pipe elements_v8 (Autodesk Fusion 360 design; units mm, degrees)
Autodesk Fusion 360 part; units mm, degrees
sketch "Esquisse1" plane through (0, 0, 0) normal (0, 0, 1) x (1, 0, 0) in component "part_1"
  circle A0 centre (0, 0) radius 12.5
  circle A1 centre (0, 0) radius 15.25
  circle A2 centre (0, 0) radius 13.5
  dimension "d1" = 25
  dimension "d2" = 30.5
  dimension "d3" = 1
  constraint coincident A0.centre A1.centre
  measures "d1" diameter of A0
  measures "d2" diameter of A1
extrude "Extrusion1" add sketch "Esquisse1" along normal blind 103 contours A2 makes body 1 in component "part_1"
extrude "Extrusion2" add sketch "Esquisse1" along normal blind 15 contours A1 bodies 1 in component "part_1"
sketch "Esquisse1 (2)" plane through (0, 0, 103) normal (0, 0, 1) x (-1, 0, 0) in component "part_2"
  circle A0 centre (0, 0) radius 12.5
  circle A1 centre (0, 0) radius 13.5
  circle A2 centre (0, 0) radius 12.5
  circle A3 centre (0, 0) radius 13.5
  circle A4 centre (0, 0) radius 15.25
extrude "Extrusion1'" add sketch "Esquisse1 (2)" along normal blind 100 separate body contours A1 A3 makes body 2 in component "part_2"
extrude "Extrusion2'" add sketch "Esquisse1 (2)" along normal blind 10 and the other way blind 10 contours A4 bodies 2 in component "part_2"
sketch "Esquisse1 (3)" plane through (0, 0, 203) normal (0, 0, 1) x (-1, 0, 0) in component "part_3"
  circle A0 centre (0, 0) radius 12.5
  circle A1 centre (0, 0) radius 13.5
  circle A2 centre (0, 0) radius 12.5
  circle A3 centre (0, 0) radius 13.5
  circle A4 centre (0, 0) radius 15.25
extrude "Extrusion1''" add sketch "Esquisse1 (3)" along normal blind 50 separate body contours A1 A3 makes body 3 in component "part_3"
extrude "Extrusion2''" add sketch "Esquisse1 (3)" along normal blind 10 and the other way blind 10 contours A4 bodies 3 in component "part_3"
sketch "Esquisse2" plane through (0, 0, 253) normal (0, 0, 1) x (-1, 0, 0) in component "part_3"
  circle A0 centre (0, 0) radius 12.5
  circle A1 centre (0, 0) radius 13.5
  circle A2 centre (0, 0) radius 15
  circle A3 centre (0, 0) radius 17
  dimension "d23" = 30
  dimension "d24" = 2
  constraint coincident A0.centre A1.centre
  measures "d23" diameter of A2
loft "Lissage1" add profiles "Esquisse2", "Esquisse1 (3)" section 1 contours A3 section 2 contours A1 A3 bodies 3 in component "part_3"
loft "Lissage2" cut profiles "Esquisse2", "Esquisse1 (3)" section 1 contours A0 | A1 | A2 section 2 contours A0 A2 bodies 3 in component "part_3"
chamfer "Chanfrein2" distance 1.75 angle 45 1 edges at (12.5864, 4.8818, 113) on bodies 2 in component "part_2"
chamfer "Chanfrein1" distance 1 angle 45 1 edges at (13.239, -5.1349, 213) on bodies 3 in component "part_3"
fillet "Congé1" radius 10 1 edges at (13.3042, -5.1602, 213.9976) on bodies 3 in component "part_3"
fillet "Congé2" radius 10 1 edges at (12.5864, -4.8818, 114.75) on bodies 2 in component "part_2"
component "part_1" placed x (1, 0, 0) y (0, 1, 0) z (0, 0, 1) at (0, 0, 0)
component "part_2" placed x (1, 0, 0) y (0, 1, 0) z (0, 0, 1) at (0, 0, 0)
component "part_3" placed x (1, 0, 0) y (0, 1, 0) z (0, 0, 1) at (0, 0, 0)
